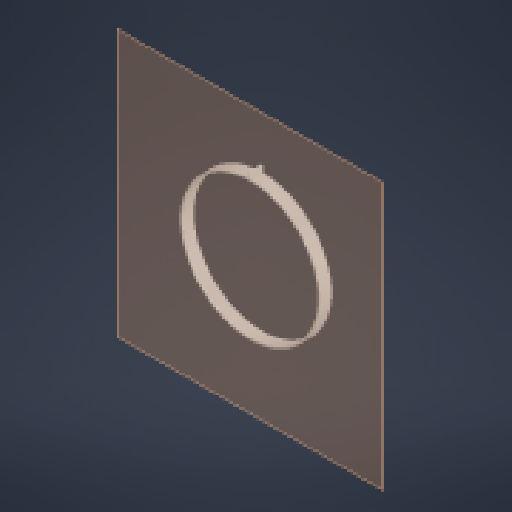
# Autodesk Inventor part: ledMount
Saved by Autodesk Inventor 2023.1 (Build 271208000, 208)
## iProperties
Created: 2023-08-24
Part Number: ledMount
Material: Generic
Document SubType Name: Modeling
Designer: washichi
Density: 1 g/cm^3
Appearance: Default
Author: washichi
Autodesk Inventor part; units mm, degrees
ref_plane "YZ Plane" through (0, 0, 0) normal (1, 0, 0) x (0, 1, 0)
ref_plane "XZ Plane" through (0, 0, 0) normal (0, 1, 0) x (-1, 0, 0)
ref_plane "XY Plane" through (0, 0, 0) normal (0, 0, 1) x (1, 0, 0)
ref_plane "Work Plane1" through (0, 0, 0) normal (0, 0, 1) x (1, 0, 0)
sketch "Sketch1" plane through (0, 0, 0) normal (0, 0, 1) x (1, 0, 0)
  circle A0 centre (0, 0) radius 85
  circle A1 centre (0, 0) radius 83
  line L0 (0, 83) -> (1, 83)
  line L1 (1, 83) -> (1, 93)
  line L2 (1, 93) -> (0, 93)
  line L3 (0, 93) -> (0, 83)
  line L4 (0, 83) -> (-1, 83)
  line L5 (-1, 83) -> (-1, 93)
  line L6 (-1, 93) -> (0, 93)
  line L7 (0, 93) -> (0, 83)
  point P0 (-1, 84.9941)
  point P1 (1, 84.9941)
  point P2 (0, 85)
  dimension "d0" = 170
  dimension "d1" = 2
  dimension "d2" = 1
  dimension "d3" = 10
  dimension "d4" = 1
  constraints: 16 end point, 4 parallel, 2 horizontal, 2 perpendicular, 1 centre point, 1 coincident, 1 point on line, 1 vertical alignment, 2 other
  measures "d0" diameter of A0
  measures "d2" distance of L2.end L1.end
  measures "d3" distance of L1.end L0.end
  measures "d4" distance of L5.end L6.end
extrude "Extrusion1" add sketch "Sketch1" against normal blind 15
body "Solid1"
